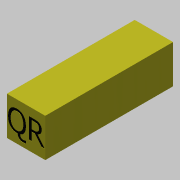
# Autodesk Inventor part: Container 2 2 5 colored color 3
Saved by Autodesk Inventor 2015 (Build 190159000, 159)
## iProperties
Created: 2015-03-07
Part Number: Container 2 2 5 colored color 3
Material: Generic
Document SubType Name: Modeling
Designer: Vukica
Density: 1 g/cm^3
Appearance: Canary
Author: Vukica
Autodesk Inventor part; units mm, degrees
ref_plane "YZ Plane" through (0, 0, 0) normal (1, 0, 0) x (0, 1, 0)
ref_plane "XZ Plane" through (0, 0, 0) normal (0, 1, 0) x (-1, 0, 0)
ref_plane "XY Plane" through (0, 0, 0) normal (0, 0, 1) x (1, 0, 0)
sketch "Sketch1" plane through (0, 0, 0) normal (0, 0, 1) x (1, 0, 0)
  line L0 (0, 0) -> (38.1, 0)
  line L1 (38.1, 0) -> (38.1, 38.1)
  line L2 (38.1, 38.1) -> (0, 38.1)
  line L3 (0, 38.1) -> (0, 0)
  dimension "d0" = 38.1
  dimension "d1" = 38.1
  constraints: 8 end point, 2 parallel, 1 horizontal, 1 perpendicular
  measures "d0" distance of L1.end L2.end
  measures "d1" distance of L2.end L0.start
extrude "Extrusion1" add sketch "Sketch1" along normal blind 127
sketch "Sketch2" plane through (0, 0, 127) normal (0, 0, 1) x (1, 0, 0)
  line L0 (-0.0121, 30.1457) -> (46.3831, 30.1457) construction
  line L1 (46.3831, 30.1457) -> (46.3831, -2.4791) construction
  line L2 (46.3831, -2.4791) -> (-0.0121, -2.4791) construction
  line L3 (-0.0121, -2.4791) -> (-0.0121, 30.1457) construction
  spline S0 degree 2 poles (18.9247, 4.4246) (18.1837, 4.2434) (16.57, 4.0458) (15.7631, 4.0458) knots 0 0 0 1 2 2 2
  spline S1 degree 2 poles (15.7631, 4.0458) (13.4742, 4.0458) (10.6255, 6.5982) (10.4937, 8.9694) knots 0 0 0 1 2 2 2
  spline S2 degree 2 poles (10.4937, 8.9694) (10.3126, 8.9694) (9.9997, 8.9694) (9.868, 8.9694) knots 0 0 0 1 2 2 2
  spline S3 degree 2 poles (9.868, 8.9694) (7.8096, 8.9694) (4.4998, 10.3691) (3.3142, 11.7358) knots 0 0 0 1 2 2 2
  spline S4 degree 2 poles (3.3142, 11.7358) (2.1451, 13.0861) (0.8936, 17.0381) (0.8936, 19.5411) knots 0 0 0 1 2 2 2
  spline S5 degree 2 poles (0.8936, 19.5411) (0.8936, 22.1099) (2.1615, 25.996) (3.3307, 27.3793) knots 0 0 0 1 2 2 2
  spline S6 degree 2 poles (3.3307, 27.3793) (4.5163, 28.746) (7.8261, 30.1457) (9.868, 30.1457) knots 0 0 0 1 2 2 2
  spline S7 degree 2 poles (9.868, 30.1457) (11.9428, 30.1457) (15.2691, 28.6966) (16.4218, 27.3793) knots 0 0 0 1 2 2 2
  spline S8 degree 2 poles (16.4218, 27.3793) (17.5744, 26.0454) (18.8588, 22.0769) (18.8588, 19.5411) knots 0 0 0 1 2 2 2
  spline S9 degree 2 poles (18.8588, 19.5411) (18.8588, 15.589) (15.7796, 10.4514) (13.0955, 9.5457) knots 0 0 0 1 2 2 2
  spline S10 degree 2 poles (13.0955, 9.5457) (13.1613, 8.7883) (13.5565, 7.5697) (13.8694, 7.2239) knots 0 0 0 1 2 2 2
  spline S11 degree 2 poles (13.8694, 7.2239) (14.2481, 6.7958) (15.2856, 6.4006) (16.2077, 6.4006) knots 0 0 0 1 2 2 2
  spline S12 degree 2 poles (16.2077, 6.4006) (16.7511, 6.4006) (18.2331, 6.7464) (18.5624, 6.8781) knots 0 0 0 1 2 2 2
  line L4 (18.5624, 6.8781) -> (18.9247, 6.8781)
  line L5 (18.9247, 6.8781) -> (18.9247, 4.4246)
  spline S13 degree 2 poles (16.043, 19.5411) (16.043, 21.5665) (15.1703, 24.6787) (14.3799, 25.6996) knots 0 0 0 1 2 2 2
  spline S14 degree 2 poles (14.3799, 25.6996) (13.573, 26.7535) (11.3006, 27.8074) (9.8844, 27.8074) knots 0 0 0 1 2 2 2
  spline S15 degree 2 poles (9.8844, 27.8074) (8.4189, 27.8074) (6.2124, 26.7864) (5.3726, 25.6996) knots 0 0 0 1 2 2 2
  spline S16 degree 2 poles (5.3726, 25.6996) (4.5657, 24.6622) (3.7094, 21.5171) (3.7094, 19.5411) knots 0 0 0 1 2 2 2
  spline S17 degree 2 poles (3.7094, 19.5411) (3.7094, 15.5396) (7.0686, 11.2747) (9.8844, 11.2747) knots 0 0 0 1 2 2 2
  spline S18 degree 2 poles (9.8844, 11.2747) (12.7003, 11.2747) (16.043, 15.5396) (16.043, 19.5411) knots 0 0 0 1 2 2 2
  line L6 (37.5486, 9.3975) -> (34.0412, 9.3975)
  line L7 (34.0412, 9.3975) -> (27.6192, 17.4827)
  line L8 (27.6192, 17.4827) -> (24.5234, 17.4827)
  line L9 (24.5234, 17.4827) -> (24.5234, 9.3975)
  line L10 (24.5234, 9.3975) -> (21.8229, 9.3975)
  line L11 (21.8229, 9.3975) -> (21.8229, 29.7175)
  line L12 (21.8229, 29.7175) -> (27.0593, 29.7175)
  spline S19 degree 2 poles (27.0593, 29.7175) (28.8048, 29.7175) (31.1595, 29.3388) (32.2299, 28.6472) knots 0 0 0 1 2 2 2
  spline S20 degree 2 poles (32.2299, 28.6472) (33.3002, 27.9556) (34.5352, 25.7984) (34.5352, 24.2012) knots 0 0 0 1 2 2 2
  spline S21 degree 2 poles (34.5352, 24.2012) (34.5352, 21.9781) (32.2628, 18.9647) (30.3197, 18.2402) knots 0 0 0 1 2 2 2
  line L13 (30.3197, 18.2402) -> (37.5486, 9.3975)
  spline S22 degree 2 poles (31.7194, 23.9871) (31.7194, 24.8763) (31.0937, 26.243) (30.435, 26.6876) knots 0 0 0 1 2 2 2
  spline S23 degree 2 poles (30.435, 26.6876) (29.8586, 27.0664) (28.3272, 27.3793) (27.2075, 27.3793) knots 0 0 0 1 2 2 2
  line L14 (27.2075, 27.3793) -> (24.5234, 27.3793)
  line L15 (24.5234, 27.3793) -> (24.5234, 19.7387)
  line L16 (24.5234, 19.7387) -> (26.8946, 19.7387)
  spline S24 degree 2 poles (26.8946, 19.7387) (28.0638, 19.7387) (29.9245, 20.1503) (30.5667, 20.7925) knots 0 0 0 1 2 2 2
  spline S25 degree 2 poles (30.5667, 20.7925) (31.1595, 21.3524) (31.7194, 22.9332) (31.7194, 23.9871) knots 0 0 0 1 2 2 2
  point P0 (0, 0)
  constraints: 2 other
extrude "Extrusion3" cut sketch "Sketch2" against normal blind 0.254
body "Solid1"
